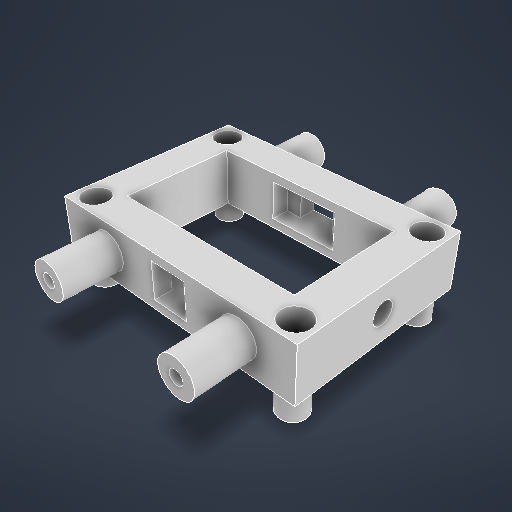
# Autodesk Inventor part: diff_gear_holder
Saved by Autodesk Inventor 2025 (Build 290162000, 162)
## iProperties
Created: 2024-07-24
Part Number: diff_gear_holder
Material: Generic
Document SubType Name: Modeling
Designer: Garfieldcmix
Density: 1 g/cm^3
Appearance: Default
Author: Garfieldcmix
Autodesk Inventor part; units mm, degrees
ref_plane "YZ Plane" through (0, 0, 0) normal (1, 0, 0) x (0, 1, 0)
ref_plane "XZ Plane" through (0, 0, 0) normal (0, 1, 0) x (-1, 0, 0)
ref_plane "XY Plane" through (0, 0, 0) normal (0, 0, 1) x (1, 0, 0)
sketch "Sketch1" plane through (0, 0, 0) normal (0, 1, 0) x (-1, 0, 0)
  line L0 (0, 0) -> (0, -39.8)
  line L1 (0, -39.8) -> (55.8, -39.8)
  line L2 (55.8, -39.8) -> (55.8, 0)
  line L3 (55.8, 0) -> (0, 0)
  line L4 (7.8, -7.8) -> (7.8, -32)
  line L5 (7.8, -32) -> (48, -32)
  line L6 (48, -32) -> (48, -7.8)
  line L7 (48, -7.8) -> (7.8, -7.8)
  line L8 (3.9, -3.9) -> (3.9, -35.9) construction
  line L9 (3.9, -35.9) -> (51.9, -35.9) construction
  line L10 (51.9, -35.9) -> (51.9, -3.9) construction
  line L11 (51.9, -3.9) -> (3.9, -3.9) construction
  circle A0 centre (3.9, -3.9) radius 1.5
  circle A1 centre (3.9, -35.9) radius 1.5
  circle A2 centre (51.9, -3.9) radius 1.5
  circle A3 centre (51.9, -35.9) radius 1.5
  circle A4 centre (3.9, -35.9) radius 3
  circle A5 centre (3.9, -3.9) radius 3
  circle A6 centre (51.9, -3.9) radius 3
  circle A7 centre (51.9, -35.9) radius 3
  dimension "d0" = 39.8
  dimension "d1" = 55.8
  dimension "d4" = 24.2
  dimension "d5" = 40.2
  dimension "d6" = 7.8
  dimension "d7" = 7.8
  dimension "d8" = 32
  dimension "d9" = 48
  dimension "d10" = 3.9
  dimension "d11" = 3.9
  dimension "d12" = 3
  dimension "d14" = 3
  dimension "d15" = 3
  dimension "d16" = 3
  dimension "d17" = 6
  dimension "d19" = 6
  dimension "d20" = 6
  dimension "d22" = 6
  constraints: 24 end point, 9 perpendicular, 8 centre point, 8 coincident, 2 parallel, 1 vertical
  measures "d0" distance of L0.start L0.end
  measures "d1" distance of L0.end L1.end
  measures "d4" distance of L4.end L4.start
  measures "d5" distance of L5.end L4.end
  measures "d6" distance between parallel lines of L1 L5
  measures "d7" distance between parallel lines of L0 L4
  measures "d8" distance of L8.start L8.end
  measures "d9" distance of L8.end L9.end
  measures "d10" distance between parallel lines of L1 L9
  measures "d11" distance between parallel lines of L0 L8
  measures "d12" diameter of A0
  measures "d14" diameter of A1
  measures "d15" diameter of A2
  measures "d16" diameter of A3
  measures "d17" diameter of A4
  measures "d19" diameter of A5
  measures "d20" diameter of A6
  measures "d22" diameter of A7
extrude "Extrusion1" add sketch "Sketch1" along normal blind 8 contours L3 L2 L1 L0
extrude "Extrusion13" add sketch "Sketch1" along normal blind 2 from surface at 8 separate body contours L3 L2 L1 L0
extrude "Extrusion12" add sketch "Sketch1" against normal blind 2 separate body contours L3 L2 L1 L0
extrude "Extrusion2" add sketch "Sketch1" along normal blind 2 from surface at -2 contours A4 | A5 | A6 | A7 bodies 1
extrude "Extrusion3" add sketch "Sketch1" against normal blind 6 from surface at -2 contours A4 | A5 | A6 | A7 bodies 1
sketch "Sketch2" plane through (0, 0, 0) normal (1, 0, 0) x (0, 0, -1)
  line L0 (0, 0) -> (0, 8) construction
  line L1 (0, 8) -> (39.8, 8) construction
  line L2 (39.8, 0) -> (39.8, 8) construction
  line L3 (0, 0) -> (39.8, 0) construction
  line L4 (0, 4) -> (39.8, 4) construction
  line L5 (19.9, 8) -> (19.9, 0) construction
  circle A0 centre (19.9, 4) radius 2.4
  dimension "d30" = 4.8
  constraints: 5 midpoint, 4 end point, 1 centre point, 1 coincident
  measures "d30" diameter of A0
extrude "Extrusion4" cut sketch "Sketch2" against normal up to surface (7.8 mm away) bodies 1
sketch "Sketch3" plane through (0, 0, -39.8) normal (0, 0, -1) x (-1, 0, 0)
  line L0 (0, 8) -> (55.8, 8) construction
  line L1 (0, 0) -> (0, 8) construction
  line L2 (0, 0) -> (55.8, 0) construction
  line L3 (55.8, 0) -> (55.8, 8) construction
  line L4 (27.9, 8) -> (27.9, 0) construction
  line L5 (0, 4) -> (55.8, 4) construction
  circle A0 centre (11.9, 4) radius 4
  circle A1 centre (11.9, 4) radius 1.5
  circle A2 centre (43.9, 4) radius 4
  circle A3 centre (43.9, 4) radius 1.5
  line L6 (20.4, 0) -> (35.4, 0)
  line L7 (35.4, 0) -> (35.4, 8)
  line L8 (35.4, 8) -> (20.4, 8)
  line L9 (20.4, 8) -> (20.4, 0)
  line L10 (27.9, 8) -> (27.9, 0) construction
  line L11 (20.4, 4) -> (35.4, 4) construction
  line L12 (23.9, 8) -> (23.9, 0)
  line L13 (31.9, 0) -> (31.9, 8)
  point P0 (27.9, 4)
  dimension "d34" = 16
  dimension "d35" = 8
  dimension "d36" = 3
  dimension "d49" = 15
  dimension "d50" = 8
  dimension "d55" = 4
  dimension "d56" = 4
  constraints: 20 end point, 10 midpoint, 5 point on line, 4 centre point, 3 coincident, 3 perpendicular, 2 parallel, 2 symmetric about line, 1 collinear, 2 other
  measures "d34" distance from line of L4 point (11.9, 4)
  measures "d35" diameter of A0
  measures "d36" diameter of A1
  measures "d49" distance of L6.start L6.end
  measures "d50" distance of L8.end L6.start
  measures "d55" distance between parallel lines of L13 L10
  measures "d56" distance between parallel lines of L12 L4
extrude "Extrusion10" cut sketch "Sketch3" against normal up to surface (7.8 mm away) contours L12 L8 L13 L6 bodies 1
extrude "Extrusion9" cut sketch "Sketch3" along normal blind 4 from surface at -7.8 contours L9 L8 L12 L6 | L13 L8 L7 L6 bodies 1
extrude "Extrusion6" add sketch "Sketch3" along normal blind 12.1 contours A0 | A2 bodies 1
sketch "Sketch4" plane through (-55.8, 0, 0) normal (0, 0, 1) x (1, 0, 0)
  line L0 (0, 8) -> (55.8, 8) construction
  line L1 (0, 0) -> (0, 8) construction
  line L2 (0, 0) -> (55.8, 0) construction
  line L3 (55.8, 0) -> (55.8, 8) construction
  line L4 (27.9, 8) -> (27.9, 0) construction
  line L5 (0, 4) -> (55.8, 4) construction
  circle A0 centre (11.9, 4) radius 4
  circle A1 centre (11.9, 4) radius 1.5
  circle A2 centre (43.9, 4) radius 4
  circle A3 centre (43.9, 4) radius 1.5
  line L6 (20.4, 0) -> (35.4, 0)
  line L7 (35.4, 0) -> (35.4, 8)
  line L8 (35.4, 8) -> (20.4, 8)
  line L9 (20.4, 8) -> (20.4, 0)
  line L10 (27.9, 8) -> (27.9, 0) construction
  line L11 (20.4, 4) -> (35.4, 4) construction
  line L12 (23.9, 8) -> (23.9, 0)
  line L13 (31.9, 0) -> (31.9, 8)
  line L14 (0, 8) -> (55.8, 8) construction
  line L15 (0, 0) -> (0, 8) construction
  line L16 (0, 0) -> (55.8, 0) construction
  line L17 (55.8, 0) -> (55.8, 8) construction
  point P0 (27.9, 4)
  dimension "d59" = 16
  dimension "d60" = 8
  dimension "d61" = 3
  dimension "d62" = 15
  dimension "d63" = 8
  dimension "d64" = 4
  dimension "d65" = 4
  constraints: 28 end point, 11 midpoint, 5 point on line, 4 centre point, 3 coincident, 3 perpendicular, 2 parallel, 2 symmetric about line, 1 collinear, 2 other
  measures "d59" distance from line of L4 point (11.9, 4)
  measures "d60" diameter of A0
  measures "d61" diameter of A1
  measures "d62" distance of L9.end L6.end
  measures "d63" distance of L9.start L9.end
  measures "d64" distance between parallel lines of L13 L10
  measures "d65" distance between parallel lines of L12 L4
extrude "Extrusion7" cut sketch "Sketch4" against normal up to surface (7.8 mm away) contours L12 L8 L13 L6 bodies 1
extrude "Extrusion11" cut sketch "Sketch4" along normal blind 4 from surface at -7.8 contours L9 L8 L12 L6 | L13 L8 L7 L6 bodies 1
extrude "Extrusion8" add sketch "Sketch4" along normal blind 12.1 contours A0 | A2 bodies 1
combine bodies "Combine1" operation type add bodies to combine 1 3 2
equation "\"d7\" = d6"
equation "\"d10\" = 0.5 * d6"
equation "\"d11\" = 0.5 * d6"
equation "\"d12\" = d14"
equation "\"d15\" = d14"
equation "\"d16\" = d14"
equation "\"d19\" = d17"
equation "\"d20\" = d21"
equation "\"d22\" = d23"
equation "\"d55\" = 0.5 * d50"
equation "\"d56\" = 0.5 * d50"
equation "\"d64\" = 0.5 * d63"
equation "\"d65\" = 0.5 * d63"
equation "\"d21\" = 6"
equation "\"d23\" = 6"
body "Solid3"
